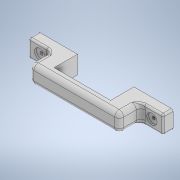
# Autodesk Inventor part: Top Bracket
Saved by Autodesk Inventor 2020 (Build 240168000, 168)
## iProperties
Created: 2019-11-12
Part Number: Top Bracket
Material: Generic
Document SubType Name: Modeling
Designer: bzs3334
Density: 1 g/cm^3
Appearance: Default
Author: bzs3334
Autodesk Inventor part; units mm, degrees
ref_plane "YZ Plane" through (0, 0, 0) normal (1, 0, 0) x (0, 1, 0)
ref_plane "XZ Plane" through (0, 0, 0) normal (0, 1, 0) x (-1, 0, 0)
ref_plane "XY Plane" through (0, 0, 0) normal (0, 0, 1) x (1, 0, 0)
sketch "Sketch1" plane through (0, 0, 0) normal (0, 1, 0) x (-1, 0, 0)
  line L0 (50, -17.5) -> (-50, -17.5)
  line L1 (-50, -17.5) -> (-50, 17.5)
  line L2 (-50, 17.5) -> (50, 17.5)
  line L3 (50, 17.5) -> (50, -17.5)
  line L4 (31.5, -17.5) -> (-31.5, -17.5)
  line L5 (-31.5, -17.5) -> (-31.5, 8.5)
  line L6 (-31.5, 8.5) -> (31.5, 8.5)
  line L7 (31.5, 8.5) -> (31.5, -17.5)
  line L8 (50, -17.5) -> (75, -17.5)
  line L9 (75, -17.5) -> (75, -6.5)
  line L10 (75, -6.5) -> (50, -6.5)
  line L11 (50, -6.5) -> (50, -17.5)
  line L12 (0, 0) -> (0, -17.5)
  line L13 (-50, -17.5) -> (-75, -17.5)
  line L14 (-75, -17.5) -> (-75, -6.5)
  line L15 (-75, -6.5) -> (-50, -6.5)
  point P0 (-31.5, -17.5)
  dimension "d0" = 100
  dimension "d1" = 50
  dimension "d2" = 35
  dimension "d3" = 17.5
  dimension "d4" = 26
  dimension "d5" = 63
  dimension "d6" = 31.5
  dimension "d7" = 11
  dimension "d8" = 25
  constraints: 32 end point, 6 parallel, 3 horizontal, 3 perpendicular, 3 symmetric about line, 1 midpoint, 1 point on line
  measures "d0" distance of L0.start L0.end
  measures "d1" distance from line of L3 L12.start
  measures "d2" distance of L2.end L0.start
  measures "d3" distance from line of L2 L12.start
  measures "d4" distance of L6.end L4.start
  measures "d5" distance of L5.end L6.end
  measures "d6" distance from line of L5 L12.start
  measures "d7" distance of L8.end L9.end
  measures "d8" distance of L9.end L10.end
extrude "Extrusion1" add sketch "Sketch1" along normal blind 20 contours L0 L7 L6 L5 L1 L2 L3 | L3 L10 L9 L8 | L13 L14 L15 L1
sketch "Sketch2" plane through (-75, 0, -6.5) normal (0, 0, 1) x (1, 0, 0)
  line L0 (0, 0) -> (25, 0) projected
  line L1 (25, 0) -> (25, 20) projected
  line L2 (0, 20) -> (25, 20) projected
  line L3 (0, 0) -> (0, 20) projected
  circle A0 centre (12.5, 10) radius 1.75
  circle A1 centre (12.5, 10) radius 5.75
  point P0 (75, 0)
  dimension "d11" = 3.5
  dimension "d12" = 11.5
  constraints: 2 centre point, 1 coincident
  measures "d11" diameter of A0
  measures "d12" diameter of A1
extrude "Extrusion2" cut sketch "Sketch2" against normal through all contours A0
extrude "Extrusion3" cut sketch "Sketch2" against normal blind 2 contours A1
mirror "Mirror1" about plane through (0, 0, 0) normal (1, 0, 0) of "Extrusion3", "Extrusion2"
fillet "Fillet1" radius 5 2 edges at (-50, 10, 17.5) (50, 10, 17.5)
fillet "Fillet2" radius 5 12 edges at (48.5355, 20, 16.0355) (50, 20, 3) (-48.5355, 20, 16.0355) (-50, 20, 3) (0, 20, 17.5) (48.5355, 0, 16.0355) (50, 0, 3) (-48.5355, 0, 16.0355) (-50, 0, 3) (0, 0, 17.5) (50, 10, -6.5) (-50, 10, -6.5)
fillet "Fillet3" radius 2 14 edges at (-75, 10, -6.5) (-48.8542, 20, -4.8773) (-64.3301, 20, -6.5) (-48.8542, 0, -4.8773) (-64.3301, 0, -6.5) (48.8542, 20, -4.8773) (64.3301, 20, -6.5) (75, 10, -6.5) (48.8542, 0, -4.8773) (64.3301, 0, -6.5) (-75, 20, -12) (-75, 0, -12) (75, 20, -12) (75, 0, -12)
equation "\"d1\" = 0.5 * d0"
equation "\"d3\" = 0.5 * d2"
equation "\"d6\" = 0.5 * d5"
body "Solid1"
